Autodesk Inventor part; units mm, degrees
(part 2 of 2)
sketch "Sketch3" plane through (-0.0003, -144.9621, -142.4319) normal (0, 0, -1) x (-1, 0, 0)
  line L0 (-10.1604, 66.049) -> (-10.1604, 136.1421) construction
  line L1 (-10.1604, 136.1421) -> (-1.0068, 136.1421) construction
  line L2 (-1.0068, 136.1421) -> (-1.0068, 66.049) construction
  line L3 (-1.0068, 66.049) -> (-10.1604, 66.049) construction
  spline S0 degree 2 poles (-7.5802, 71.9161) (-7.0615, 71.9161) (-6.128, 71.5465) (-5.8038, 71.2159) knots 0 0 0 1 2 2 2
  spline S1 degree 2 poles (-5.8038, 71.2159) (-5.3954, 70.801) (-4.974, 69.6794) (-4.974, 68.8237) knots 0 0 0 1 2 2 2
  line L4 (-4.974, 68.8237) -> (-4.974, 67.9225)
  line L5 (-4.974, 67.9225) -> (-1.9918, 67.9225)
  line L6 (-1.9918, 67.9225) -> (-1.9918, 66.8593)
  line L7 (-1.9918, 66.8593) -> (-9.9918, 66.8593)
  line L8 (-9.9918, 66.8593) -> (-9.9918, 68.8691)
  spline S2 degree 2 poles (-9.9918, 68.8691) (-9.9918, 69.5822) (-9.7585, 70.5806) (-9.4927, 70.9631) knots 0 0 0 1 2 2 2
  spline S3 degree 2 poles (-9.4927, 70.9631) (-9.188, 71.4104) (-8.2479, 71.9161) (-7.5802, 71.9161) knots 0 0 0 1 2 2 2
  spline S4 degree 2 poles (-7.5478, 70.8075) (-7.9627, 70.8075) (-8.5721, 70.5222) (-8.7666, 70.2305) knots 0 0 0 1 2 2 2
  spline S5 degree 2 poles (-8.7666, 70.2305) (-8.9351, 69.9777) (-9.0713, 69.3034) (-9.0713, 68.8042) knots 0 0 0 1 2 2 2
  line L9 (-9.0713, 68.8042) -> (-9.0713, 67.9225)
  line L10 (-9.0713, 67.9225) -> (-5.8816, 67.9225)
  line L11 (-5.8816, 67.9225) -> (-5.8816, 68.6486)
  spline S6 degree 2 poles (-5.8816, 68.6486) (-5.8816, 69.2969) (-6.0891, 70.0943) (-6.3614, 70.3537) knots 0 0 0 1 2 2 2
  spline S7 degree 2 poles (-6.3614, 70.3537) (-6.6012, 70.5935) (-7.1653, 70.8075) (-7.5478, 70.8075) knots 0 0 0 1 2 2 2
  line L12 (-1.9918, 79.1187) -> (-1.9918, 77.7378)
  line L13 (-1.9918, 77.7378) -> (-5.175, 75.2094)
  line L14 (-5.175, 75.2094) -> (-5.175, 73.9906)
  line L15 (-5.175, 73.9906) -> (-1.9918, 73.9906)
  line L16 (-1.9918, 73.9906) -> (-1.9918, 72.9274)
  line L17 (-1.9918, 72.9274) -> (-9.9918, 72.9274)
  line L18 (-9.9918, 72.9274) -> (-9.9918, 74.989)
  spline S8 degree 2 poles (-9.9918, 74.989) (-9.9918, 75.6762) (-9.8427, 76.6033) (-9.5705, 77.0247) knots 0 0 0 1 2 2 2
  spline S9 degree 2 poles (-9.5705, 77.0247) (-9.2982, 77.446) (-8.4489, 77.9323) (-7.82, 77.9323) knots 0 0 0 1 2 2 2
  spline S10 degree 2 poles (-7.82, 77.9323) (-6.9448, 77.9323) (-5.7585, 77.0376) (-5.4732, 76.2726) knots 0 0 0 1 2 2 2
  line L19 (-5.4732, 76.2726) -> (-1.9918, 79.1187)
  spline S11 degree 2 poles (-7.7358, 76.8237) (-8.0858, 76.8237) (-8.6239, 76.5773) (-8.799, 76.318) knots 0 0 0 1 2 2 2
  spline S12 degree 2 poles (-8.799, 76.318) (-8.9481, 76.0911) (-9.0713, 75.4882) (-9.0713, 75.0473) knots 0 0 0 1 2 2 2
  line L20 (-9.0713, 75.0473) -> (-9.0713, 73.9906)
  line L21 (-9.0713, 73.9906) -> (-6.0632, 73.9906)
  line L22 (-6.0632, 73.9906) -> (-6.0632, 74.9242)
  spline S13 degree 2 poles (-6.0632, 74.9242) (-6.0632, 75.3845) (-6.2252, 76.117) (-6.4781, 76.3699) knots 0 0 0 1 2 2 2
  spline S14 degree 2 poles (-6.4781, 76.3699) (-6.6985, 76.6033) (-7.3209, 76.8237) (-7.7358, 76.8237) knots 0 0 0 1 2 2 2
  spline S15 degree 2 poles (-9.0777, 85.4136) (-8.5461, 85.8674) (-6.9902, 86.3731) (-5.9918, 86.3731) knots 0 0 0 1 2 2 2
  spline S16 degree 2 poles (-5.9918, 86.3731) (-5.0194, 86.3731) (-3.444, 85.8804) (-2.9124, 85.4136) knots 0 0 0 1 2 2 2
  spline S17 degree 2 poles (-2.9124, 85.4136) (-2.3549, 84.9209) (-1.8233, 83.6178) (-1.8233, 82.8334) knots 0 0 0 1 2 2 2
  spline S18 degree 2 poles (-1.8233, 82.8334) (-1.8233, 82.023) (-2.3743, 80.7264) (-2.9124, 80.2532) knots 0 0 0 1 2 2 2
  spline S19 degree 2 poles (-2.9124, 80.2532) (-3.444, 79.7929) (-5.0064, 79.3002) (-5.9918, 79.3002) knots 0 0 0 1 2 2 2
  spline S20 degree 2 poles (-5.9918, 79.3002) (-6.9967, 79.3002) (-8.5267, 79.7994) (-9.0777, 80.2597) knots 0 0 0 1 2 2 2
  spline S21 degree 2 poles (-9.0777, 80.2597) (-9.6094, 80.7264) (-10.1604, 82.0295) (-10.1604, 82.8334) knots 0 0 0 1 2 2 2
  spline S22 degree 2 poles (-10.1604, 82.8334) (-10.1604, 83.6503) (-9.5899, 84.9598) (-9.0777, 85.4136) knots 0 0 0 1 2 2 2
  spline S23 degree 2 poles (-5.9918, 85.2645) (-6.7828, 85.2645) (-8.0081, 84.9209) (-8.41, 84.6097) knots 0 0 0 1 2 2 2
  spline S24 degree 2 poles (-8.41, 84.6097) (-8.8249, 84.2921) (-9.2398, 83.3974) (-9.2398, 82.8399) knots 0 0 0 1 2 2 2
  spline S25 degree 2 poles (-9.2398, 82.8399) (-9.2398, 82.2629) (-8.8379, 81.3942) (-8.41, 81.0636) knots 0 0 0 1 2 2 2
  spline S26 degree 2 poles (-8.41, 81.0636) (-8.0016, 80.7459) (-6.7698, 80.4088) (-5.9918, 80.4088) knots 0 0 0 1 2 2 2
  spline S27 degree 2 poles (-5.9918, 80.4088) (-4.4165, 80.4088) (-2.7439, 81.7313) (-2.7439, 82.8399) knots 0 0 0 1 2 2 2
  spline S28 degree 2 poles (-2.7439, 82.8399) (-2.7439, 83.9485) (-4.4165, 85.2645) (-5.9918, 85.2645) knots 0 0 0 1 2 2 2
  line L23 (-1.9918, 89.4071) -> (-9.0453, 89.4071)
  line L24 (-9.0453, 89.4071) -> (-9.0453, 86.7232)
  line L25 (-9.0453, 86.7232) -> (-9.9918, 86.7232)
  line L26 (-9.9918, 86.7232) -> (-9.9918, 93.1543)
  line L27 (-9.9918, 93.1543) -> (-9.0453, 93.1543)
  line L28 (-9.0453, 93.1543) -> (-9.0453, 90.4704)
  line L29 (-9.0453, 90.4704) -> (-1.9918, 90.4704)
  line L30 (-1.9918, 90.4704) -> (-1.9918, 89.4071)
  spline S29 degree 2 poles (-9.0777, 99.6243) (-8.5461, 100.0781) (-6.9902, 100.5838) (-5.9918, 100.5838) knots 0 0 0 1 2 2 2
  spline S30 degree 2 poles (-5.9918, 100.5838) (-5.0194, 100.5838) (-3.444, 100.0911) (-2.9124, 99.6243) knots 0 0 0 1 2 2 2
  spline S31 degree 2 poles (-2.9124, 99.6243) (-2.3549, 99.1316) (-1.8233, 97.8285) (-1.8233, 97.0441) knots 0 0 0 1 2 2 2
  spline S32 degree 2 poles (-1.8233, 97.0441) (-1.8233, 96.2337) (-2.3743, 94.9371) (-2.9124, 94.4639) knots 0 0 0 1 2 2 2
  spline S33 degree 2 poles (-2.9124, 94.4639) (-3.444, 94.0036) (-5.0064, 93.5109) (-5.9918, 93.5109) knots 0 0 0 1 2 2 2
  spline S34 degree 2 poles (-5.9918, 93.5109) (-6.9967, 93.5109) (-8.5267, 94.0101) (-9.0777, 94.4704) knots 0 0 0 1 2 2 2
  spline S35 degree 2 poles (-9.0777, 94.4704) (-9.6094, 94.9371) (-10.1604, 96.2402) (-10.1604, 97.0441) knots 0 0 0 1 2 2 2
  spline S36 degree 2 poles (-10.1604, 97.0441) (-10.1604, 97.861) (-9.5899, 99.1705) (-9.0777, 99.6243) knots 0 0 0 1 2 2 2
  spline S37 degree 2 poles (-5.9918, 99.4752) (-6.7828, 99.4752) (-8.0081, 99.1316) (-8.41, 98.8204) knots 0 0 0 1 2 2 2
  spline S38 degree 2 poles (-8.41, 98.8204) (-8.8249, 98.5028) (-9.2398, 97.6081) (-9.2398, 97.0506) knots 0 0 0 1 2 2 2
  spline S39 degree 2 poles (-9.2398, 97.0506) (-9.2398, 96.4736) (-8.8379, 95.6049) (-8.41, 95.2742) knots 0 0 0 1 2 2 2
  spline S40 degree 2 poles (-8.41, 95.2742) (-8.0016, 94.9566) (-6.7698, 94.6195) (-5.9918, 94.6195) knots 0 0 0 1 2 2 2
  spline S41 degree 2 poles (-5.9918, 94.6195) (-4.4165, 94.6195) (-2.7439, 95.942) (-2.7439, 97.0506) knots 0 0 0 1 2 2 2
  spline S42 degree 2 poles (-2.7439, 97.0506) (-2.7439, 98.1592) (-4.4165, 99.4752) (-5.9918, 99.4752) knots 0 0 0 1 2 2 2
  line L31 (-1.9918, 103.6178) -> (-9.0453, 103.6178)
  line L32 (-9.0453, 103.6178) -> (-9.0453, 100.9339)
  line L33 (-9.0453, 100.9339) -> (-9.9918, 100.9339)
  line L34 (-9.9918, 100.9339) -> (-9.9918, 107.365)
  line L35 (-9.9918, 107.365) -> (-9.0453, 107.365)
  line L36 (-9.0453, 107.365) -> (-9.0453, 104.6811)
  line L37 (-9.0453, 104.6811) -> (-1.9918, 104.6811)
  line L38 (-1.9918, 104.6811) -> (-1.9918, 103.6178)
  line L39 (-9.9918, 113.7767) -> (-5.5316, 111.0733)
  line L40 (-5.5316, 111.0733) -> (-1.9918, 111.0733)
  line L41 (-1.9918, 111.0733) -> (-1.9918, 110.0101)
  line L42 (-1.9918, 110.0101) -> (-5.4213, 110.0101)
  line L43 (-5.4213, 110.0101) -> (-9.9918, 107.3067)
  line L44 (-9.9918, 107.3067) -> (-9.9918, 108.4866)
  line L45 (-9.9918, 108.4866) -> (-6.4716, 110.5482)
  line L46 (-6.4716, 110.5482) -> (-9.9918, 112.6486)
  line L47 (-9.9918, 112.6486) -> (-9.9918, 113.7767)
  spline S43 degree 2 poles (-7.5802, 119.5725) (-7.0615, 119.5725) (-6.128, 119.2029) (-5.8038, 118.8723) knots 0 0 0 1 2 2 2
  spline S44 degree 2 poles (-5.8038, 118.8723) (-5.3954, 118.4574) (-4.974, 117.3358) (-4.974, 116.4801) knots 0 0 0 1 2 2 2
  line L48 (-4.974, 116.4801) -> (-4.974, 115.5789)
  line L49 (-4.974, 115.5789) -> (-1.9918, 115.5789)
  line L50 (-1.9918, 115.5789) -> (-1.9918, 114.5157)
  line L51 (-1.9918, 114.5157) -> (-9.9918, 114.5157)
  line L52 (-9.9918, 114.5157) -> (-9.9918, 116.5255)
  spline S45 degree 2 poles (-9.9918, 116.5255) (-9.9918, 117.2386) (-9.7585, 118.237) (-9.4927, 118.6195) knots 0 0 0 1 2 2 2
  spline S46 degree 2 poles (-9.4927, 118.6195) (-9.188, 119.0668) (-8.2479, 119.5725) (-7.5802, 119.5725) knots 0 0 0 1 2 2 2
  spline S47 degree 2 poles (-7.5478, 118.4639) (-7.9627, 118.4639) (-8.5721, 118.1786) (-8.7666, 117.8869) knots 0 0 0 1 2 2 2
  spline S48 degree 2 poles (-8.7666, 117.8869) (-8.9351, 117.6341) (-9.0713, 116.9598) (-9.0713, 116.4606) knots 0 0 0 1 2 2 2
  line L53 (-9.0713, 116.4606) -> (-9.0713, 115.5789)
  line L54 (-9.0713, 115.5789) -> (-5.8816, 115.5789)
  line L55 (-5.8816, 115.5789) -> (-5.8816, 116.305)
  spline S49 degree 2 poles (-5.8816, 116.305) (-5.8816, 116.9533) (-6.0891, 117.7507) (-6.3614, 118.0101) knots 0 0 0 1 2 2 2
  spline S50 degree 2 poles (-6.3614, 118.0101) (-6.6012, 118.2499) (-7.1653, 118.4639) (-7.5478, 118.4639) knots 0 0 0 1 2 2 2
  line L56 (-1.9918, 120.5838) -> (-9.9918, 120.5838)
  line L57 (-9.9918, 120.5838) -> (-9.9918, 125.5887)
  line L58 (-9.9918, 125.5887) -> (-9.0453, 125.5887)
  line L59 (-9.0453, 125.5887) -> (-9.0453, 121.647)
  line L60 (-9.0453, 121.647) -> (-6.8541, 121.647)
  line L61 (-6.8541, 121.647) -> (-6.8541, 125.3229)
  line L62 (-6.8541, 125.3229) -> (-5.9076, 125.3229)
  line L63 (-5.9076, 125.3229) -> (-5.9076, 121.647)
  line L64 (-5.9076, 121.647) -> (-2.9384, 121.647)
  line L65 (-2.9384, 121.647) -> (-2.9384, 125.5887)
  line L66 (-2.9384, 125.5887) -> (-1.9918, 125.5887)
  line L67 (-1.9918, 125.5887) -> (-1.9918, 120.5838)
  line L68 (-1.9918, 134.4963) -> (-1.9918, 130.5935)
  line L69 (-1.9918, 130.5935) -> (-2.8087, 130.5935)
  line L70 (-2.8087, 130.5935) -> (-2.8087, 132.0457)
  line L71 (-2.8087, 132.0457) -> (-8.1701, 132.0457)
  line L72 (-8.1701, 132.0457) -> (-8.1701, 130.5935)
  line L73 (-8.1701, 130.5935) -> (-8.9027, 130.5935)
  spline S51 degree 2 poles (-8.9027, 130.5935) (-8.9027, 131.4169) (-9.3695, 132.1948) (-10.0178, 132.2467) knots 0 0 0 1 2 2 2
  line L74 (-10.0178, 132.2467) -> (-10.0178, 133.0765)
  line L75 (-10.0178, 133.0765) -> (-2.8087, 133.0765)
  line L76 (-2.8087, 133.0765) -> (-2.8087, 134.4963)
  line L77 (-2.8087, 134.4963) -> (-1.9918, 134.4963)
  point P0 (-0.0003, 144.9621)
  constraints: 2 other
extrude "Extrusion3" add sketch "Sketch3" against normal blind 2
ref_plane "Work Plane4" through (-0.0003, -144.9621, 0) normal (-0.0000018, -1, 0) x (-0.0015858, 0, -0.9999987)
sketch "Sketch4" plane through (-0.0003, -144.9621, 0) normal (-0.0000018, -1, 0) x (-0.0015858, 0, -0.9999987)
  line L0 (16.9921, 58.4768) -> (58.7681, 58.4768) construction
  line L1 (58.7681, 58.4768) -> (58.7681, 41.9273) construction
  line L2 (58.7681, 41.9273) -> (16.9921, 41.9273) construction
  line L3 (16.9921, 41.9273) -> (16.9921, 58.4768) construction
  line L4 (19.5835, 52.3699) -> (17.2593, 52.3699)
  line L5 (17.2593, 52.3699) -> (17.2593, 52.9825)
  line L6 (17.2593, 52.9825) -> (18.0227, 52.9825)
  line L7 (18.0227, 52.9825) -> (18.0227, 57.7572)
  line L8 (18.0227, 57.7572) -> (17.2593, 57.7572)
  line L9 (17.2593, 57.7572) -> (17.2593, 58.3699)
  line L10 (17.2593, 58.3699) -> (19.5835, 58.3699)
  line L11 (19.5835, 58.3699) -> (19.5835, 57.7572)
  line L12 (19.5835, 57.7572) -> (18.8201, 57.7572)
  line L13 (18.8201, 57.7572) -> (18.8201, 52.9825)
  line L14 (18.8201, 52.9825) -> (19.5835, 52.9825)
  line L15 (19.5835, 52.9825) -> (19.5835, 52.3699)
  line L16 (24.8639, 52.3699) -> (23.9692, 52.3699)
  line L17 (23.9692, 52.3699) -> (21.3144, 57.5433)
  line L18 (21.3144, 57.5433) -> (21.3144, 52.3699)
  line L19 (21.3144, 52.3699) -> (20.5705, 52.3699)
  line L20 (20.5705, 52.3699) -> (20.5705, 58.3699)
  line L21 (20.5705, 58.3699) -> (21.7034, 58.3699)
  line L22 (21.7034, 58.3699) -> (24.12, 53.6195)
  line L23 (24.12, 53.6195) -> (24.12, 58.3699)
  line L24 (24.12, 58.3699) -> (24.8639, 58.3699)
  line L25 (24.8639, 58.3699) -> (24.8639, 52.3699)
  line L26 (27.4798, 52.3699) -> (27.4798, 57.66)
  line L27 (27.4798, 57.66) -> (25.4668, 57.66)
  line L28 (25.4668, 57.66) -> (25.4668, 58.3699)
  line L29 (25.4668, 58.3699) -> (30.2901, 58.3699)
  line L30 (30.2901, 58.3699) -> (30.2901, 57.66)
  line L31 (30.2901, 57.66) -> (28.2772, 57.66)
  line L32 (28.2772, 57.66) -> (28.2772, 52.3699)
  line L33 (28.2772, 52.3699) -> (27.4798, 52.3699)
  line L34 (30.8979, 52.3699) -> (30.8979, 58.3699)
  line L35 (30.8979, 58.3699) -> (34.6516, 58.3699)
  line L36 (34.6516, 58.3699) -> (34.6516, 57.66)
  line L37 (34.6516, 57.66) -> (31.6953, 57.66)
  line L38 (31.6953, 57.66) -> (31.6953, 56.0165)
  line L39 (31.6953, 56.0165) -> (34.4522, 56.0165)
  line L40 (34.4522, 56.0165) -> (34.4522, 55.3067)
  line L41 (34.4522, 55.3067) -> (31.6953, 55.3067)
  line L42 (31.6953, 55.3067) -> (31.6953, 53.0797)
  line L43 (31.6953, 53.0797) -> (34.6516, 53.0797)
  line L44 (34.6516, 53.0797) -> (34.6516, 52.3699)
  line L45 (34.6516, 52.3699) -> (30.8979, 52.3699)
  line L46 (40.1702, 52.3699) -> (39.1345, 52.3699)
  line L47 (39.1345, 52.3699) -> (37.2383, 54.7572)
  line L48 (37.2383, 54.7572) -> (36.3242, 54.7572)
  line L49 (36.3242, 54.7572) -> (36.3242, 52.3699)
  line L50 (36.3242, 52.3699) -> (35.5268, 52.3699)
  line L51 (35.5268, 52.3699) -> (35.5268, 58.3699)
  line L52 (35.5268, 58.3699) -> (37.073, 58.3699)
  spline S0 degree 2 poles (37.073, 58.3699) (37.5883, 58.3699) (38.2836, 58.258) (38.5997, 58.0538) knots 0 0 0 1 2 2 2
  spline S1 degree 2 poles (38.5997, 58.0538) (38.9157, 57.8496) (39.2804, 57.2126) (39.2804, 56.741) knots 0 0 0 1 2 2 2
  spline S2 degree 2 poles (39.2804, 56.741) (39.2804, 56.0846) (38.6094, 55.1948) (38.0357, 54.9809) knots 0 0 0 1 2 2 2
  line L53 (38.0357, 54.9809) -> (40.1702, 52.3699)
  spline S3 degree 2 poles (38.449, 56.6778) (38.449, 56.9404) (38.2642, 57.3439) (38.0697, 57.4752) knots 0 0 0 1 2 2 2
  spline S4 degree 2 poles (38.0697, 57.4752) (37.8995, 57.587) (37.4473, 57.6794) (37.1167, 57.6794) knots 0 0 0 1 2 2 2
  line L54 (37.1167, 57.6794) -> (36.3242, 57.6794)
  line L55 (36.3242, 57.6794) -> (36.3242, 55.4233)
  line L56 (36.3242, 55.4233) -> (37.0243, 55.4233)
  spline S5 degree 2 poles (37.0243, 55.4233) (37.3695, 55.4233) (37.919, 55.5449) (38.1086, 55.7345) knots 0 0 0 1 2 2 2
  spline S6 degree 2 poles (38.1086, 55.7345) (38.2836, 55.8998) (38.449, 56.3666) (38.449, 56.6778) knots 0 0 0 1 2 2 2
  line L57 (44.235, 57.66) -> (41.4441, 57.66)
  line L58 (41.4441, 57.66) -> (41.4441, 55.9679)
  line L59 (41.4441, 55.9679) -> (44.1183, 55.9679)
  line L60 (44.1183, 55.9679) -> (44.1183, 55.258)
  line L61 (44.1183, 55.258) -> (41.4441, 55.258)
  line L62 (41.4441, 55.258) -> (41.4441, 52.3699)
  line L63 (41.4441, 52.3699) -> (40.6467, 52.3699)
  line L64 (40.6467, 52.3699) -> (40.6467, 58.3699)
  line L65 (40.6467, 58.3699) -> (44.235, 58.3699)
  line L66 (44.235, 58.3699) -> (44.235, 57.66)
  line L67 (44.3031, 52.3699) -> (46.3258, 58.3699)
  line L68 (46.3258, 58.3699) -> (47.308, 58.3699)
  line L69 (47.308, 58.3699) -> (49.3307, 52.3699)
  line L70 (49.3307, 52.3699) -> (48.4895, 52.3699)
  line L71 (48.4895, 52.3699) -> (47.9449, 54.0473)
  line L72 (47.9449, 54.0473) -> (45.6548, 54.0473)
  line L73 (45.6548, 54.0473) -> (45.1102, 52.3699)
  line L74 (45.1102, 52.3699) -> (44.3031, 52.3699)
  line L75 (47.7261, 54.728) -> (46.7974, 57.553)
  line L76 (46.7974, 57.553) -> (45.8736, 54.728)
  line L77 (45.8736, 54.728) -> (47.7261, 54.728)
  spline S7 degree 2 poles (52.2431, 52.2629) (51.6597, 52.2629) (50.6726, 52.6567) (50.3128, 53.0506) knots 0 0 0 1 2 2 2
  spline S8 degree 2 poles (50.3128, 53.0506) (49.953, 53.4396) (49.5592, 54.6065) (49.5592, 55.365) knots 0 0 0 1 2 2 2
  spline S9 degree 2 poles (49.5592, 55.365) (49.5592, 56.1186) (49.9433, 57.237) (50.308, 57.6503) knots 0 0 0 1 2 2 2
  spline S10 degree 2 poles (50.308, 57.6503) (50.6678, 58.0538) (51.6499, 58.4768) (52.2577, 58.4768) knots 0 0 0 1 2 2 2
  spline S11 degree 2 poles (52.2577, 58.4768) (52.5592, 58.4768) (53.0892, 58.3893) (53.3128, 58.3212) knots 0 0 0 1 2 2 2
  spline S12 degree 2 poles (53.3128, 58.3212) (53.5073, 58.258) (53.9109, 58.0781) (54.1102, 57.9712) knots 0 0 0 1 2 2 2
  line L78 (54.1102, 57.9712) -> (54.1102, 57.0084)
  line L79 (54.1102, 57.0084) -> (54.047, 57.0084)
  spline S13 degree 2 poles (54.047, 57.0084) (53.9401, 57.1057) (53.6094, 57.378) (53.3712, 57.5092) knots 0 0 0 1 2 2 2
  spline S14 degree 2 poles (53.3712, 57.5092) (53.1426, 57.6357) (52.6029, 57.7961) (52.2529, 57.7961) knots 0 0 0 1 2 2 2
  spline S15 degree 2 poles (52.2529, 57.7961) (51.8687, 57.7961) (51.1832, 57.4801) (50.9255, 57.1786) knots 0 0 0 1 2 2 2
  spline S16 degree 2 poles (50.9255, 57.1786) (50.6726, 56.8723) (50.3906, 55.9436) (50.3906, 55.365) knots 0 0 0 1 2 2 2
  spline S17 degree 2 poles (50.3906, 55.365) (50.3906, 54.7475) (50.6872, 53.8577) (50.9449, 53.5514) knots 0 0 0 1 2 2 2
  spline S18 degree 2 poles (50.9449, 53.5514) (51.1978, 53.2548) (51.8736, 52.9533) (52.2529, 52.9533) knots 0 0 0 1 2 2 2
  spline S19 degree 2 poles (52.2529, 52.9533) (52.5981, 52.9533) (53.1864, 53.1235) (53.4149, 53.2499) knots 0 0 0 1 2 2 2
  spline S20 degree 2 poles (53.4149, 53.2499) (53.6337, 53.3763) (53.9595, 53.6389) (54.0519, 53.7313) knots 0 0 0 1 2 2 2
  line L80 (54.0519, 53.7313) -> (54.1102, 53.7313)
  line L81 (54.1102, 53.7313) -> (54.1102, 52.7783)
  spline S21 degree 2 poles (54.1102, 52.7783) (53.9109, 52.6859) (53.5608, 52.5157) (53.3128, 52.4379) knots 0 0 0 1 2 2 2
  spline S22 degree 2 poles (53.3128, 52.4379) (53.0503, 52.3504) (52.6029, 52.2629) (52.2431, 52.2629) knots 0 0 0 1 2 2 2
  line L82 (54.8542, 52.3699) -> (54.8542, 58.3699)
  line L83 (54.8542, 58.3699) -> (58.6078, 58.3699)
  line L84 (58.6078, 58.3699) -> (58.6078, 57.66)
  line L85 (58.6078, 57.66) -> (55.6516, 57.66)
  line L86 (55.6516, 57.66) -> (55.6516, 56.0165)
  line L87 (55.6516, 56.0165) -> (58.4084, 56.0165)
  line L88 (58.4084, 56.0165) -> (58.4084, 55.3067)
  line L89 (58.4084, 55.3067) -> (55.6516, 55.3067)
  line L90 (55.6516, 55.3067) -> (55.6516, 53.0797)
  line L91 (55.6516, 53.0797) -> (58.6078, 53.0797)
  line L92 (58.6078, 53.0797) -> (58.6078, 52.3699)
  line L93 (58.6078, 52.3699) -> (54.8542, 52.3699)
  line L94 (27.6621, 42.491) -> (26.8647, 42.491)
  line L95 (26.8647, 42.491) -> (26.8647, 47.6596)
  line L96 (26.8647, 47.6596) -> (25.299, 44.1442)
  line L97 (25.299, 44.1442) -> (24.8128, 44.1442)
  line L98 (24.8128, 44.1442) -> (23.2618, 47.6596)
  line L99 (23.2618, 47.6596) -> (23.2618, 42.491)
  line L100 (23.2618, 42.491) -> (22.5178, 42.491)
  line L101 (22.5178, 42.491) -> (22.5178, 48.491)
  line L102 (22.5178, 48.491) -> (23.607, 48.491)
  line L103 (23.607, 48.491) -> (25.1046, 45.1507)
  line L104 (25.1046, 45.1507) -> (26.5535, 48.491)
  line L105 (26.5535, 48.491) -> (27.6621, 48.491)
  line L106 (27.6621, 48.491) -> (27.6621, 42.491)
  spline S23 degree 2 poles (33.1224, 47.8054) (33.4627, 47.4067) (33.842, 46.2398) (33.842, 45.491) knots 0 0 0 1 2 2 2
  spline S24 degree 2 poles (33.842, 45.491) (33.842, 44.7617) (33.4725, 43.5802) (33.1224, 43.1815) knots 0 0 0 1 2 2 2
  spline S25 degree 2 poles (33.1224, 43.1815) (32.7529, 42.7633) (31.7755, 42.3646) (31.1872, 42.3646) knots 0 0 0 1 2 2 2
  spline S26 degree 2 poles (31.1872, 42.3646) (30.5794, 42.3646) (29.607, 42.7779) (29.252, 43.1815) knots 0 0 0 1 2 2 2
  spline S27 degree 2 poles (29.252, 43.1815) (28.9068, 43.5802) (28.5373, 44.752) (28.5373, 45.491) knots 0 0 0 1 2 2 2
  spline S28 degree 2 poles (28.5373, 45.491) (28.5373, 46.2447) (28.9117, 47.3922) (29.2569, 47.8054) knots 0 0 0 1 2 2 2
  spline S29 degree 2 poles (29.2569, 47.8054) (29.607, 48.2041) (30.5843, 48.6174) (31.1872, 48.6174) knots 0 0 0 1 2 2 2
  spline S30 degree 2 poles (31.1872, 48.6174) (31.7999, 48.6174) (32.782, 48.1896) (33.1224, 47.8054) knots 0 0 0 1 2 2 2
  spline S31 degree 2 poles (33.0106, 45.491) (33.0106, 46.0842) (32.7529, 47.0032) (32.5195, 47.3046) knots 0 0 0 1 2 2 2
  spline S32 degree 2 poles (32.5195, 47.3046) (32.2812, 47.6158) (31.6102, 47.927) (31.1921, 47.927) knots 0 0 0 1 2 2 2
  spline S33 degree 2 poles (31.1921, 47.927) (30.7593, 47.927) (30.1078, 47.6255) (29.8598, 47.3046) knots 0 0 0 1 2 2 2
  spline S34 degree 2 poles (29.8598, 47.3046) (29.6216, 46.9983) (29.3687, 46.0745) (29.3687, 45.491) knots 0 0 0 1 2 2 2
  spline S35 degree 2 poles (29.3687, 45.491) (29.3687, 44.3095) (30.3606, 43.055) (31.1921, 43.055) knots 0 0 0 1 2 2 2
  spline S36 degree 2 poles (31.1921, 43.055) (32.0235, 43.055) (33.0106, 44.3095) (33.0106, 45.491) knots 0 0 0 1 2 2 2
  spline S37 degree 2 poles (39.4482, 45.4862) (39.4482, 44.6644) (38.782, 43.3419) (38.2229, 42.9724) knots 0 0 0 1 2 2 2
  spline S38 degree 2 poles (38.2229, 42.9724) (37.7658, 42.6855) (36.8274, 42.491) (36.0981, 42.491) knots 0 0 0 1 2 2 2
  line L107 (36.0981, 42.491) -> (34.7172, 42.491)
  line L108 (34.7172, 42.491) -> (34.7172, 48.491)
  line L109 (34.7172, 48.491) -> (36.0835, 48.491)
  spline S39 degree 2 poles (36.0835, 48.491) (36.9295, 48.491) (37.8922, 48.2382) (38.2326, 48.0145) knots 0 0 0 1 2 2 2
  spline S40 degree 2 poles (38.2326, 48.0145) (38.8112, 47.6304) (39.4482, 46.3614) (39.4482, 45.4862) knots 0 0 0 1 2 2 2
  spline S41 degree 2 poles (38.6167, 45.4959) (38.6167, 46.1863) (38.1597, 47.1636) (37.7075, 47.4408) knots 0 0 0 1 2 2 2
  spline S42 degree 2 poles (37.7075, 47.4408) (37.3866, 47.6304) (36.6621, 47.8006) (36.1224, 47.8006) knots 0 0 0 1 2 2 2
  line L110 (36.1224, 47.8006) -> (35.5146, 47.8006)
  line L111 (35.5146, 47.8006) -> (35.5146, 43.1815)
  line L112 (35.5146, 43.1815) -> (36.1224, 43.1815)
  spline S43 degree 2 poles (36.1224, 43.1815) (36.6524, 43.1815) (37.4546, 43.3516) (37.7804, 43.5802) knots 0 0 0 1 2 2 2
  spline S44 degree 2 poles (37.7804, 43.5802) (38.1986, 43.8622) (38.6167, 44.7957) (38.6167, 45.4959) knots 0 0 0 1 2 2 2
  spline S45 degree 2 poles (42.4093, 42.3646) (41.8793, 42.3646) (41.0916, 42.6417) (40.8144, 42.9189) knots 0 0 0 1 2 2 2
  spline S46 degree 2 poles (40.8144, 42.9189) (40.4984, 43.2301) (40.2407, 44.1053) (40.2407, 44.7471) knots 0 0 0 1 2 2 2
  line L113 (40.2407, 44.7471) -> (40.2407, 48.491)
  line L114 (40.2407, 48.491) -> (41.0381, 48.491)
  line L115 (41.0381, 48.491) -> (41.0381, 44.7471)
  spline S47 degree 2 poles (41.0381, 44.7471) (41.0381, 44.3289) (41.1451, 43.7649) (41.2958, 43.5364) knots 0 0 0 1 2 2 2
  spline S48 degree 2 poles (41.2958, 43.5364) (41.4563, 43.2933) (42.0106, 43.0453) (42.4093, 43.0453) knots 0 0 0 1 2 2 2
  spline S49 degree 2 poles (42.4093, 43.0453) (42.7837, 43.0453) (43.3671, 43.2933) (43.5276, 43.5364) knots 0 0 0 1 2 2 2
  spline S50 degree 2 poles (43.5276, 43.5364) (43.6783, 43.7649) (43.7853, 44.3241) (43.7853, 44.7276) knots 0 0 0 1 2 2 2
  line L116 (43.7853, 44.7276) -> (43.7853, 48.491)
  line L117 (43.7853, 48.491) -> (44.5827, 48.491)
  line L118 (44.5827, 48.491) -> (44.5827, 44.7471)
  spline S51 degree 2 poles (44.5827, 44.7471) (44.5827, 44.1199) (44.3298, 43.2252) (44.0089, 42.9189) knots 0 0 0 1 2 2 2
  spline S52 degree 2 poles (44.0089, 42.9189) (43.7221, 42.6369) (42.9636, 42.3646) (42.4093, 42.3646) knots 0 0 0 1 2 2 2
  line L119 (49.2018, 42.491) -> (45.7253, 42.491)
  line L120 (45.7253, 42.491) -> (45.7253, 48.491)
  line L121 (45.7253, 48.491) -> (46.5227, 48.491)
  line L122 (46.5227, 48.491) -> (46.5227, 43.2009)
  line L123 (46.5227, 43.2009) -> (49.2018, 43.2009)
  line L124 (49.2018, 43.2009) -> (49.2018, 42.491)
  line L125 (49.829, 42.491) -> (49.829, 48.491)
  line L126 (49.829, 48.491) -> (53.5827, 48.491)
  line L127 (53.5827, 48.491) -> (53.5827, 47.7811)
  line L128 (53.5827, 47.7811) -> (50.6264, 47.7811)
  line L129 (50.6264, 47.7811) -> (50.6264, 46.1377)
  line L130 (50.6264, 46.1377) -> (53.3833, 46.1377)
  line L131 (53.3833, 46.1377) -> (53.3833, 45.4278)
  line L132 (53.3833, 45.4278) -> (50.6264, 45.4278)
  line L133 (50.6264, 45.4278) -> (50.6264, 43.2009)
  line L134 (50.6264, 43.2009) -> (53.5827, 43.2009)
  line L135 (53.5827, 43.2009) -> (53.5827, 42.491)
  line L136 (53.5827, 42.491) -> (49.829, 42.491)
  point P0 (0, 0)
  constraints: 2 other
extrude "Extrusion4" add sketch "Sketch4" against normal blind 2
body "Solid1"
